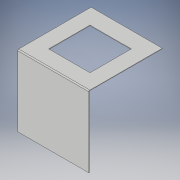
# Autodesk Inventor part: Part1
Saved by Autodesk Inventor 2019 (Build 230136000, 136)
## iProperties
Created: 2019-12-05
Part Number: Part1
Material: Generic
Document SubType Name: Sheet Metal
Designer: User
Density: 1 g/cm^3
Sheet Metal Rule: Default
Appearance: Default
Author: User
Autodesk Inventor part; units mm, degrees
ref_plane "YZ Plane" through (0, 0, 0) normal (1, 0, 0) x (0, 1, 0)
ref_plane "XZ Plane" through (0, 0, 0) normal (0, 1, 0) x (-1, 0, 0)
ref_plane "XY Plane" through (0, 0, 0) normal (0, 0, 1) x (1, 0, 0)
sketch "Sketch1" plane through (0, 0, 0) normal (0, 1, 0) x (-1, 0, 0)
  line L0 (-49.2125, 50.8) -> (49.2125, 50.8)
  line L1 (49.2125, 50.8) -> (49.2125, -50.8)
  line L2 (49.2125, -50.8) -> (-49.2125, -50.8)
  line L3 (-49.2125, -50.8) -> (-49.2125, 50.8)
  line L4 (-49.2125, 50.8) -> (49.2125, -50.8) construction
  line L5 (49.2125, 50.8) -> (-49.2125, -50.8) construction
  point P0 (0, 0)
  dimension "d0" = 98.425
  dimension "d1" = 101.6
  measures "d0" distance of L1.end L2.end
  measures "d1" distance of L0.end L1.end
extrude "Plate1" add sketch "Sketch1" along normal blind 0.7144
sketch "Sketch2" plane through (-49.2125, 0.7144, 50.0856) normal (0, 0, 1) x (1, 0, 0)
  line L0 (98.425, 0) -> (0, 0)
  line L1 (0, 0) -> (0, -98.425)
  line L2 (0, -98.425) -> (98.425, -98.425)
  line L3 (98.425, -98.425) -> (98.425, 0)
  constraints: 6 end point, 1 horizontal, 1 perpendicular, 1 vertical
edge flange "Flange1" height 98.425 angle 90 thickness 0.7144 bend radius 0.7144 thickness toward (0, 0, 1) relief tear relief width 0.7144 relief depth 0.3572 edges at (0, 0, 50.8) wall of the first edge with corners at (49.2125, 0.7144, 50.0856) (-49.2125, 0.7144, 50.0856) (-49.2125, -97.7106, 50.0856) (49.2125, -97.7106, 50.0856)
bend "Bend1"
corner "Corner1"
sketch "Sketch3" plane through (0, 0.7144, 0) normal (0, 1, 0) x (1, 0, 0)
  line L0 (28.575, -28.575) -> (-28.575, -28.575)
  line L1 (-28.575, -28.575) -> (-28.575, 28.575)
  line L2 (-28.575, 28.575) -> (28.575, 28.575)
  line L3 (28.575, 28.575) -> (28.575, -28.575)
  line L4 (28.575, -28.575) -> (-28.575, 28.575) construction
  line L5 (-28.575, -28.575) -> (28.575, 28.575) construction
  point P0 (0, 0)
  dimension "d13" = 57.15
  dimension "d14" = 57.15
  constraints: 12 end point, 2 midpoint, 2 parallel, 1 horizontal, 1 perpendicular
  measures "d13" distance of L1.end L2.end
  measures "d14" distance of L0.end L1.end
extrude "Extrusion1" cut sketch "Sketch3" against normal blind 0.7144
equation "\"d15\" = Thickness"
equation "\"d2\" = Thickness"
equation "\"d3\" = BendReliefWidth"
equation "\"d4\" = BendReliefDepth"
equation "\"d5\" = MinimumRemnant"
equation "\"d6\" = TransitionRadius"
equation "\"d9\" = BendRadius"
equation "\"d10\" = CornerReliefSize"
equation "\"d11\" = GapSize"
equation "\"d12\" = JacobiRadiusSize"
equation "\"BendRadius\" = Thickness"
equation "\"BendReliefWidth\" = Thickness"
equation "\"BendReliefDepth\" = 0.5 * Thickness"
equation "\"CornerReliefSize\" = 4 * Thickness"
equation "\"MinimumRemnant\" = 2 * Thickness"
equation "\"TransitionRadius\" = BendRadius"
equation "\"JacobiRadiusSize\" = BendRadius"
equation "\"GapSize\" = Thickness"
equation "\"Thickness\" = 0.714375"
body "Solid1"
